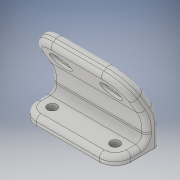
# Autodesk Inventor part: SwitchMount
Saved by Autodesk Inventor 2017 (Build 210142000, 142)
## iProperties
Created: 2017-09-15
Part Number: SwitchMount
Material: Generic
Document SubType Name: Modeling
Designer: Axel
Density: 1 g/cm^3
Appearance: Default
Author: Axel
Autodesk Inventor part; units mm, degrees
ref_plane "YZ Plane" through (0, 0, 0) normal (1, 0, 0) x (0, 1, 0)
ref_plane "XZ Plane" through (0, 0, 0) normal (0, 1, 0) x (-1, 0, 0)
ref_plane "XY Plane" through (0, 0, 0) normal (0, 0, 1) x (1, 0, 0)
sketch "Sketch5" plane through (0, 0, 0) normal (1, 0, 0) x (0, 1, 0)
  line L0 (0, 0) -> (0, 14)
  line L1 (0, 14) -> (3, 14)
  line L2 (3, 14) -> (3, 4)
  line L3 (3, 4) -> (8.8859, 4)
  line L4 (8.8859, 4) -> (21.9322, 11.8789)
  line L5 (21.9322, 11.8789) -> (24, 8.4549)
  line L6 (24, 8.4549) -> (10, 0)
  line L7 (10, 0) -> (0, 0)
  dimension "d31" = 3
  dimension "d32" = 4
  dimension "d33" = 4
  dimension "d34" = 14
  dimension "d35" = 10
  dimension "d36" = 10
  constraints: 16 end point, 5 perpendicular, 1 parallel, 1 vertical
  measures "d31" distance between parallel lines of L2 L0
  measures "d32" distance between parallel lines of L7 L3
  measures "d33" distance between parallel lines of L6 L4
  measures "d34" horizontal distance of L6.end L5.end
  measures "d35" distance of L0.start L6.end
  measures "d36" vertical distance of L2.end L0.end
extrude "Extrusion4" add sketch "Sketch5" along normal blind 30
sketch "Sketch6" plane through (0, 3, 14) normal (0, 1, 0) x (1, 0, 0)
  circle A0 centre (5, 5) radius 1.5
  circle A1 centre (25, 5) radius 1.5
  line L0 (30, 10) -> (30, 0) projected
  line L1 (0, 0) -> (30, 0) projected
  line L2 (0, 0) -> (0, 10) projected
  point P0 (0, 14)
  dimension "d39" = 3
  dimension "d40" = 3
  dimension "d41" = 5
  dimension "d42" = 5
  dimension "d43" = 5
  dimension "d44" = 5
  constraints: 2 centre point
  measures "d39" diameter of A0
  measures "d40" diameter of A1
  measures "d41" distance from line of L0 A1.centre
  measures "d42" distance from line of L1 A1.centre
  measures "d43" distance from line of L2 A0.centre
  measures "d44" distance from line of L1 A0.centre
extrude "Extrusion5" cut sketch "Sketch6" against normal blind 30
fillet "Fillet5" radius 5 2 edges at (0, 1.5, 14) (30, 1.5, 14)
sketch "Sketch7" plane through (30, 24, 8.4549) normal (0, 0.517, -0.856) x (-1, 0, 0)
  arc A0 (8.5, -9) -> (5.5, -9) centre (7, -7) ccw
  arc A1 (24.5, -9) -> (21.5, -9) centre (23, -7) ccw
  line L0 (30, 0) -> (30, -16.355) projected
  line L1 (30, 0) -> (0, 0) projected
  line L2 (0, -16.355) -> (0, 0) projected
  line L3 (5.5, -9) -> (8.5, -9)
  line L4 (21.5, -9) -> (24.5, -9)
  point P0 (30, -24.9151)
  dimension "d48" = 5
  dimension "d49" = 5
  dimension "d50" = 7
  dimension "d51" = 7
  dimension "d52" = 7
  dimension "d53" = 7
  dimension "d54" = 4.5
  constraints: 4 end point, 4 point on circle, 2 centre point, 2 point on line, 1 horizontal
  measures "d48" diameter of A0
  measures "d49" diameter of A1
  measures "d50" distance from line of L0 A1.centre
  measures "d51" distance from line of L1 A1.centre
  measures "d52" distance from line of L1 A0.centre
  measures "d53" distance from line of L2 A0.centre
extrude "Extrusion6" cut sketch "Sketch7" against normal blind 30
fillet "Fillet6" radius 7 2 edges at (0, 22.9661, 10.1669) (30, 22.9661, 10.1669)
sketch "Sketch8" plane through (0, 8.8859, 4) normal (0, -0.517, 0.856) x (1, 0, 0)
  arc A0 (8.5, 6.2408) -> (5.5, 6.2408) centre (7, 8.2408) ccw projected
  circle A1 centre (7, 8.2408) radius 3.25
  arc A2 (24.5, 6.2408) -> (21.5, 6.2408) centre (23, 8.2408) ccw projected
  circle A3 centre (23, 8.2408) radius 3.25
  point P0 (0, -9.6742)
  dimension "d58" = 6.5
  dimension "d59" = 6.5
  constraints: 2 centre point, 2 coincident
  measures "d58" diameter of A1
  measures "d59" diameter of A3
extrude "Extrusion7" cut sketch "Sketch8" against normal blind 0.8
fillet "Fillet7" radius 2 1 edges at (15, 3, 4)
fillet "Fillet8" radius 12 2 edges at (15, 8.8859, 4) (15, 10, 0)
fillet "Fillet9" radius 1.5 9 edges at (15, 24, 8.4549) (2.0503, 22.245, 7.395) (0, 15.4345, 3.282) (0, 9.8774, 0.44) (0, 3.3288, 0) (30, 15.4345, 3.282) (30, 9.8774, 0.44) (30, 3.3288, 0) (27.9497, 22.245, 7.395)
fillet "Fillet10" radius 1.5 14 edges at (30, 13.8435, 6.9941) (27.9497, 20.1771, 10.819) (15, 21.9322, 11.8789) (2.0503, 20.1771, 10.819) (0, 13.8435, 6.9941) (0, 8.7633, 4.44) (0, 5.2717, 4) (0, 3, 7.5) (1.4645, 3, 12.5355) (15, 3, 14) (28.5355, 3, 12.5355) (30, 3, 7.5) (30, 5.2717, 4) (30, 8.7633, 4.44)
fillet "Fillet11" radius 0.5 8 edges at (29.5607, 0, 0.4393) (15, 0, 0) (0.4393, 0, 0.4393) (0, 0, 5.25) (1.4645, 0, 12.5355) (15, 0, 14) (28.5355, 0, 12.5355) (30, 0, 5.25)
body "Solid2"
